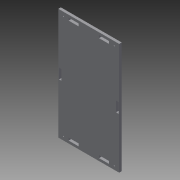
# Autodesk Inventor part: basePanel01
Saved by Autodesk Inventor 2013 (Build 170138000, 138)
## iProperties
Created: 2014-10-07
Part Number: basePanel01
Material: Generic
Document SubType Name: Modeling
Designer: Nano
Density: 1 g/cm^3
Author: Nano
Autodesk Inventor part; units mm, degrees
ref_plane "YZ Plane" through (0, 0, 0) normal (1, 0, 0) x (0, 1, 0)
ref_plane "XZ Plane" through (0, 0, 0) normal (0, 1, 0) x (-1, 0, 0)
ref_plane "XY Plane" through (0, 0, 0) normal (0, 0, 1) x (1, 0, 0)
sketch "Sketch1" plane through (0, 0, 0) normal (0, 0, 1) x (1, 0, 0)
  line L0 (0, -12.7) -> (0, 266.7) projected
  line L1 (-152.4, 266.7) -> (-152.4, -12.7) projected
  line L2 (0, 266.7) -> (-152.4, 266.7) projected
  line L3 (-152.4, -12.7) -> (0, -12.7) projected
  line L4 (-126.6434, 0) -> (-126.6434, -6.35) projected
  line L5 (-126.6434, -6.35) -> (-101.2434, -6.35) projected
  line L6 (-101.2434, -6.35) -> (-101.2434, 0) projected
  line L7 (-101.2434, 0) -> (-126.6434, 0) projected
  line L8 (-50.4434, 0) -> (-50.4434, -6.35) projected
  line L9 (-50.4434, -6.35) -> (-25.0434, -6.35) projected
  line L10 (-25.0434, -6.35) -> (-25.0434, 0) projected
  line L11 (-25.0434, 0) -> (-50.4434, 0) projected
  line L12 (-126.6434, 260.35) -> (-126.6434, 254) projected
  line L13 (-126.6434, 254) -> (-101.2434, 254) projected
  line L14 (-101.2434, 254) -> (-101.2434, 260.35) projected
  line L15 (-101.2434, 260.35) -> (-126.6434, 260.35) projected
  line L16 (-50.4434, 260.35) -> (-50.4434, 254) projected
  line L17 (-50.4434, 254) -> (-25.0434, 254) projected
  line L18 (-25.0434, 254) -> (-25.0434, 260.35) projected
  line L19 (-25.0434, 260.35) -> (-50.4434, 260.35) projected
  circle A0 centre (-12.7, 257.175) radius 1.8542 projected
  circle A1 centre (-139.7, 257.175) radius 1.8542 projected
  circle A2 centre (-139.7, -3.175) radius 1.8542 projected
  circle A3 centre (-12.7, -3.175) radius 1.8542 projected
  point P0 (0, 0)
extrude "Extrusion1" add sketch "Sketch1" along normal blind 6.35
sketch "Sketch2" plane through (0, 0, 6.35) normal (0, 0, 1) x (1, 0, 0)
  line L0 (-150.8125, 139.7) -> (-144.4625, 139.7) projected
  line L1 (-150.8125, 114.3) -> (-150.8125, 139.7) projected
  line L2 (-144.4625, 114.3) -> (-150.8125, 114.3) projected
  line L3 (-144.4625, 139.7) -> (-144.4625, 114.3) projected
  line L4 (-7.9375, 139.7) -> (-1.5875, 139.7) projected
  line L5 (-7.9375, 114.3) -> (-7.9375, 139.7) projected
  line L6 (-1.5875, 114.3) -> (-7.9375, 114.3) projected
  line L7 (-1.5875, 139.7) -> (-1.5875, 114.3) projected
  point P0 (0, 0)
extrude "Extrusion2" cut sketch "Sketch2" against normal through all
body "Solid1"
